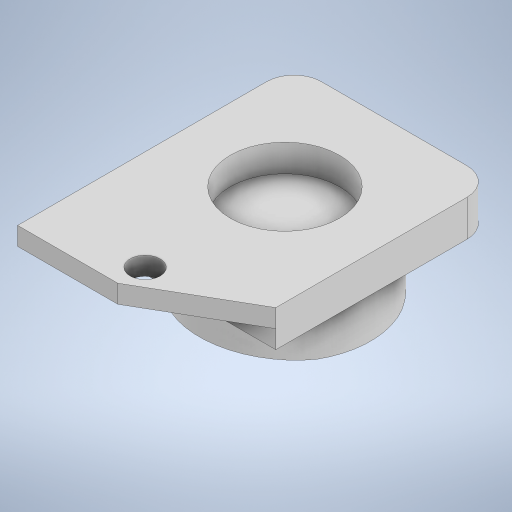
# Autodesk Inventor part: bracket_2
Saved by Autodesk Inventor 2024.3 (Build 283343000, 343)
## iProperties
Created: 2025-10-03
Part Number: bracket_2
Material: 일반
Document SubType Name: Modeling
Designer: joung
Density: 1 g/cm^3
Appearance: 기본값
Author: joung
Autodesk Inventor part; units mm, degrees
ref_plane "YZ Plane" through (0, 0, 0) normal (1, 0, 0) x (0, 1, 0)
ref_plane "XZ Plane" through (0, 0, 0) normal (0, 1, 0) x (-1, 0, 0)
ref_plane "XY Plane" through (0, 0, 0) normal (0, 0, 1) x (1, 0, 0)
sketch "스케치1" plane through (0, 0, 0) normal (0, 1, 0) x (-1, 0, 0)
  circle A0 centre (0, 0) radius 47
  circle A1 centre (0, 0) radius 35
  line L0 (0, 0) -> (0, 145.5)
  circle A2 centre (0, 145.5) radius 48.5
  circle A3 centre (0, 145.5) radius 36.5
  dimension "d0" = 94
  dimension "d1" = 12
  dimension "d2" = 145.5
  dimension "d3" = 97
  dimension "d4" = 12
  constraints: 4 centre point, 2 coincident, 2 end point, 1 vertical
  measures "d0" diameter of A0
  measures "d1" radial gap between concentric circles of A0 A1
  measures "d2" distance of L0.start L0.end
  measures "d3" diameter of A2
  measures "d4" radial gap between concentric circles of A2 A3
extrude "돌출1" add sketch "스케치1" along normal blind 30 contours A0
sketch "스케치2" plane through (0, 30, 0) normal (0, 1, 0) x (1, 0, 0)
  line L0 (-55, 60) -> (55, 60)
  line L1 (55, 60) -> (55, -60)
  line L2 (55, -60) -> (-55, -60)
  line L3 (-55, -60) -> (-55, 60)
  line L4 (-55, 60) -> (55, -60) construction
  line L5 (55, 60) -> (-55, -60) construction
  point P0 (0, 0)
  dimension "d7" = 110
  dimension "d8" = 120
  constraints: 12 end point, 2 midpoint, 2 parallel, 1 horizontal, 1 perpendicular
  measures "d7" distance of L1.end L2.end
  measures "d8" distance of L0.end L1.end
extrude "돌출2" add sketch "스케치2" along normal blind 20
fillet "모깎기1" radius 15 2 edges at (-55, 40, -60) (55, 40, -60)
sketch "스케치5" plane through (0, 50, 0) normal (0, 1, 0) x (1, 0, 0)
  circle A0 centre (0, 0) radius 30
  circle A1 centre (0, 0) radius 38
  dimension "d22" = 60
  dimension "d23" = 8
  constraints: 2 centre point, 1 coincident
  measures "d22" diameter of A0
  measures "d23" radial gap between concentric circles of A0 A1
extrude "돌출5" [suppressed]
sketch "스케치6" plane through (0, 50, 0) normal (0, 1, 0) x (1, 0, 0)
  circle A0 centre (0, 0) radius 30
  constraints: 1 centre point, 1 coincident
extrude "돌출6" cut sketch "스케치6" against normal blind 15
sketch "스케치7" plane through (0, 50, 0) normal (0, 1, 0) x (1, 0, 0)
  line L0 (-55, 45) -> (-55, -60) projected
  line L1 (-55, -60) -> (0, -91.7543)
  line L2 (-55, -60) -> (8.5085, -60) construction
  line L3 (55, -60) -> (55, 45) projected
  line L4 (0, -91.7543) -> (55, -60)
  line L5 (0, -91.7543) -> (0, -76.7543)
  circle A0 centre (0, -76.7543) radius 8.25
  line L6 (-55, -60) -> (55, -60)
  point P0 (0, 0)
  dimension "d28" = 30
  dimension "d29" = 15
  dimension "d30" = 16.5
  constraints: 10 end point, 2 horizontal, 1 centre point, 1 coincident, 1 equal length, 1 vertical
  measures "d28" angle of L1 L2
  measures "d29" distance of L1.end L5.end
  measures "d30" diameter of A0
extrude "돌출7" add sketch "스케치7" against normal blind 10
fillet "모깎기2" radius 5 1 edges at (0, 45, 91.7543)
sketch "스케치8" plane through (0, 0, 0) normal (0, -1, 0) x (1, 0, 0)
  circle A0 centre (0, 0) radius 35
  constraints: 1 centre point, 1 coincident
extrude "돌출8" add sketch "스케치8" against normal up to surface (30 mm away)
sketch "스케치9" plane through (0, 0, 0) normal (1, 0, 0) x (0, 1, 0)
  line L0 (0, -47) -> (0, 47) projected
  line L1 (0, 0) -> (0, 47)
  line L2 (0, 47) -> (0, 23.5)
  line L3 (0, 23.5) -> (2.056, 47)
  line L4 (0, 47) -> (30, 47) projected
  line L5 (0, 23.5) -> (23.5898, 23.5) construction
  line L6 (0, 0) -> (0, -47)
  line L7 (0, -23.5) -> (2.056, -47)
  line L8 (0, -47) -> (2.056, -47)
  dimension "d36" = 85
  constraints: 14 end point, 2 horizontal, 2 midpoint, 2 vertical, 1 equal length, 1 point on line
  measures "d36" angle of L5 L3
extrude "돌출9" cut sketch "스케치9" along normal mid plane 100
sketch "스케치10" plane through (0, 50, 0) normal (0, 1, 0) x (1, 0, 0)
  line L0 (-55, -60) -> (-2.5, -90.3109) projected
  line L1 (-55, -60) -> (-2.5, -90.3109)
  line L2 (-2.5, -90.3109) -> (0, -91.7543)
  line L3 (0, -91.7543) -> (-55, -91.7543)
  line L4 (-55, -91.7543) -> (-55, -60)
  line L5 (55, -60) -> (2.5, -90.3109) projected
  line L6 (0, -91.7543) -> (2.5, -90.3109)
  arc A0 (-2.5, -90.3109) -> (2.5, -90.3109) centre (0, -85.9808) ccw projected
  circle A1 centre (0, -85.9808) radius 5
  point P0 (0, 0)
  dimension "d41" = 31.7543
  dimension "d42" = 55
  dimension "d43" = 60.6218
  constraints: 10 end point, 2 collinear, 1 centre point, 1 coincident, 1 horizontal, 1 perpendicular, 1 point on line
  measures "d41" distance of L3.end L0.start
  measures "d42" distance of L2.end L3.end
  measures "d43" distance of L0.start L0.end
extrude "돌출10" add sketch "스케치10" against normal up to surface (10 mm away) contours L0 L2 L3 L4 | A0 L6 L2
